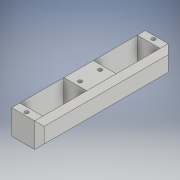
# Autodesk Inventor part: FEMUR2_A
Saved by Autodesk Inventor 2017 (Build 210142000, 142)
## iProperties
Created: 2017-09-24
Part Number: FEMUR2_A
Material: Generic
Document SubType Name: Modeling
Designer: Alexander Miller
Density: 1 g/cm^3
Appearance: Default
Author: Alexander Miller
Autodesk Inventor part; units mm, degrees
ref_plane "YZ Plane" through (0, 0, 0) normal (1, 0, 0) x (0, 1, 0)
ref_plane "XZ Plane" through (0, 0, 0) normal (0, 1, 0) x (-1, 0, 0)
ref_plane "XY Plane" through (0, 0, 0) normal (0, 0, 1) x (1, 0, 0)
sketch "Sketch1" plane through (0, 0, 0) normal (0, 1, 0) x (-1, 0, 0)
  line L0 (35, -8.5) -> (-35, -8.5)
  line L1 (-35, -8.5) -> (-35, 8.5)
  line L2 (-35, 8.5) -> (35, 8.5)
  line L3 (35, 8.5) -> (35, -8.5)
  point P0 (0, 0)
  point P1 (0, -8.5)
  point P2 (35, 0)
  dimension "d0" = 70
  dimension "d1" = 17
  constraints: 8 end point, 2 midpoint, 2 parallel, 1 horizontal, 1 horizontal alignment, 1 perpendicular, 1 vertical alignment
  measures "d0" distance of L0.start L0.end
  measures "d1" distance of L2.end L0.start
extrude "Extrusion1" add sketch "Sketch1" along normal blind 13
sketch "Sketch2" plane through (0, 13, 0) normal (0, 1, 0) x (1, 0, 0)
  line L0 (-30.75, 6) -> (-7.75, 6)
  line L1 (-7.75, 6) -> (-7.75, -6)
  line L2 (-7.75, -6) -> (-30.75, -6)
  line L3 (-30.75, -6) -> (-30.75, 6)
  circle A0 centre (-33.25, 0) radius 1
  circle A1 centre (-5.25, 0) radius 1
  line L4 (0, 11.9) -> (0, -11.9) construction
  line L5 (-35, 8.5) -> (-35, -8.5) projected
  line L6 (30.75, 6) -> (7.75, 6)
  line L7 (7.75, 6) -> (7.75, -6)
  line L8 (7.75, -6) -> (30.75, -6)
  line L9 (30.75, -6) -> (30.75, 6)
  circle A2 centre (33.25, 0) radius 1
  circle A3 centre (5.25, 0) radius 1
  point P0 (0, 0)
  point P1 (-7.75, 0)
  dimension "d4" = 23
  dimension "d5" = 12
  dimension "d6" = 2
  dimension "d7" = 1.5
  dimension "d8" = 1.5
  dimension "d9" = 4.25
  constraints: 16 end point, 6 symmetric about line, 4 centre point, 3 horizontal alignment, 2 parallel, 1 equal radius, 1 horizontal, 1 midpoint, 1 perpendicular, 2 other
  measures "d4" distance of L0.start L0.end
  measures "d5" distance of L2.end L0.start
  measures "d6" diameter of A0
  measures "d7" distance edge to line of A0 L3
  measures "d8" distance edge to line of A1 L1
  measures "d9" distance between parallel lines of L5 L3
extrude "Extrusion2" cut sketch "Sketch2" against normal through all
chamfer "Chamfer1" distance 2.5 angle 45 4 edges at (-35, 6.5, 8.5) (-35, 6.5, -8.5) (35, 6.5, 8.5) (35, 6.5, -8.5)
chamfer "Chamfer2" distance 2.5 angle 45 4 edges at (0, 13, -8.5) (0, 13, 8.5) (0, 0, 8.5) (0, 0, -8.5)
equation "\"d4\" = servo_A"
equation "\"d5\" = servo_B"
equation "\"d6\" = servo_H"
equation "\"d7\" = servo_L"
equation "\"d8\" = servo_L"
equation "\"d9\" = -0.5 * servo_A + 0.5 * servo_D"
equation "\"servo_A\" = 23"
equation "\"servo_B\" = 12"
equation "\"servo_H\" = 2"
equation "\"servo_L\" = 1.5"
equation "\"servo_D\" = 31.5"
body "Solid1"
